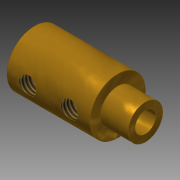
# Autodesk Inventor part: Vtulka
Saved by Autodesk Inventor 2014 (Build 180170000, 170)
## iProperties
Created: 2017-11-13
Part Number: Vtulka
Material: Типовые
Document SubType Name: Modeling
Designer: Nikopol
Density: 1 g/cm^3
Appearance: Сварка — латунь
Author: Nikopol
Autodesk Inventor part; units mm, degrees
ref_plane "YZ Plane" through (0, 0, 0) normal (1, 0, 0) x (0, 1, 0)
ref_plane "XY Plane" through (0, 0, 0) normal (0, 0, 1) x (1, 0, 0)
sketch "Эскиз1" plane through (0, 0, 0) normal (1, 0, 0) x (0, 1, 0)
  circle A0 centre (0, 0) radius 1.5
  circle A1 centre (0, 0) radius 4
  dimension "d0" = 3
  dimension "d1" = 8
  constraints: 2 centre point, 2 coincident
  measures "d0" diameter of A0
  measures "d1" diameter of A1
extrude "Выдавливание1" add sketch "Эскиз1" along normal blind 12
sketch "Эскиз2" plane through (12, 0, 0) normal (1, 0, 0) x (0, 0, -1)
  circle A0 centre (0, 0) radius 1.5 projected
  circle A1 centre (0, 0) radius 4 projected
  circle A2 centre (0, 0) radius 2.5
  dimension "d4" = 5
  constraints: 1 centre point, 1 coincident
  measures "d4" diameter of A2
extrude "Выдавливание2" add sketch "Эскиз2" along normal blind 4 contours A2
ref_plane "РабПлоскость1" through (0, -4, 0) normal (0, 1, 0) x (-1, 0, 0)
sketch "Эскиз3" plane through (0, -4, 0) normal (0, 1, 0) x (-1, 0, 0)
  point P0 (0, 0)
  point P1 (-3, 0)
  point P2 (-9, 0)
  dimension "d7" = 3
  dimension "d8" = 6
  measures "d7" distance of point (-3, 0) point (0, 0)
  measures "d8" distance of point (-9, 0) point (-3, 0)
hole "Отверстие1" at (3, -4, 0) at (9, -4, 0) direction (0, 1, 0) diameter 2.459 depth 3 tip angle 118 thread size "M3x0.5" class "6H" standard "ISO Metric profile"
